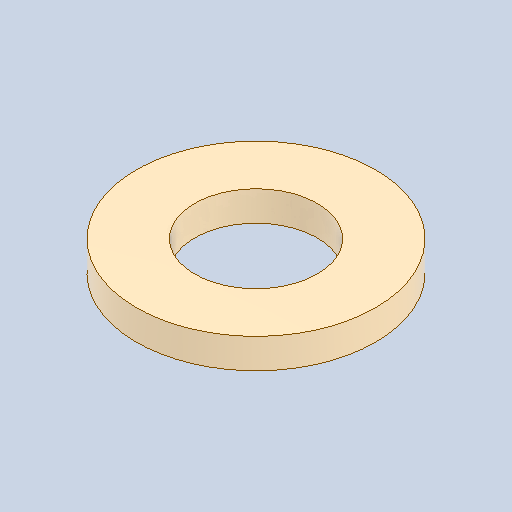
# Autodesk Inventor part: ceramic_washer_M4_v1
Saved by Autodesk Inventor 2026.2 (Build 302298000, 298)
## iProperties
Created: 2019-11-08
Part Number: ceramic_washer_M4_v1
Material: Silicon Nitride
Document SubType Name: Modeling
Designer: kuzmin
Density: 3.18 g/cm^3
Appearance: Smooth - Off-White
Mass: 0.13382 g
Surface Area: 1.30675 cm^2
Volume: 0.0420816 cm^3
Author: kuzmin
Autodesk Inventor part; units mm, degrees
ref_plane "YZ Plane" through (0, 0, 0) normal (1, 0, 0) x (0, 1, 0)
ref_plane "XZ Plane" through (0, 0, 0) normal (0, 1, 0) x (-1, 0, 0)
ref_plane "XY Plane" through (0, 0, 0) normal (0, 0, 1) x (1, 0, 0)
sketch "Sketch1" plane through (0, 0, 0) normal (0, 0, 1) x (1, 0, 0)
  line L0 (4, 0) -> (4, 1)
  line L1 (4, 1) -> (2.05, 1)
  line L2 (2.05, 1) -> (2.05, 0)
  line L3 (0, 0) -> (0, 8.8913)
  line L4 (2.05, 0) -> (4, 0)
  dimension "d2" = 1
  dimension "d3" = 4.1
  dimension "d4" = 8
  constraints: 10 end point, 1 horizontal, 1 perpendicular, 1 vertical
  measures "d2" distance of L0.start L0.end
  measures "d3" diameter of L2 L3
  measures "d4" diameter of L0 L3
revolve "Revolution1" add sketch "Sketch1" angle 360 about axis through (0, 0, 0) along (0, 1, 0)
equation "\"d2\" = t1"
equation "\"d3\" = id"
equation "\"d4\" = od_a"
equation "\"od_a\" = 8"
equation "\"t1\" = 1"
equation "\"id\" = 4.1"
body "Solid1"
